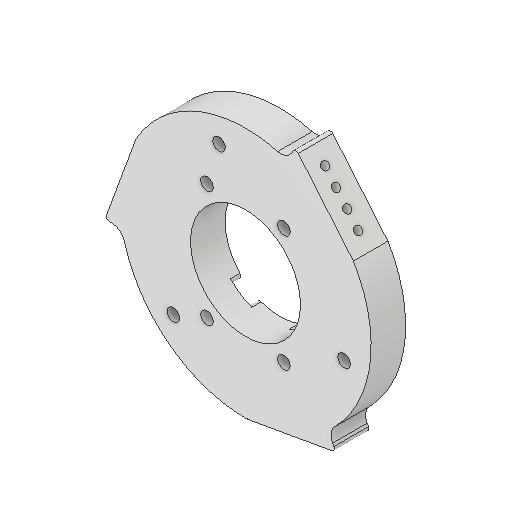
# Autodesk Inventor part: 3DP_ABS_Bowl_Feeder_Base_Plate
Saved by Autodesk Inventor 2025 (Build 290162010, 162A)
## iProperties
Created: 2018-05-26
Part Number: 3DP_ABS_Bowl_Feeder_Base_Plate
Material: ABS Plastic
Document SubType Name: Modeling
Designer: Andrzej
Density: 1.06 g/cm^3
Appearance: Smooth - White
Author: Andrzej
Autodesk Inventor part; units mm, degrees
ref_plane "YZ Plane" through (0, 0, 0) normal (1, 0, 0) x (0, 1, 0)
ref_plane "XZ Plane" through (0, 0, 0) normal (0, 1, 0) x (-1, 0, 0)
ref_plane "XY Plane" through (0, 0, 0) normal (0, 0, 1) x (1, 0, 0)
sketch "Sketch1" plane through (0, 0, 0) normal (0, 0, 1) x (1, 0, 0)
  circle A0 centre (0, 0) radius 40
  circle A1 centre (0, 0) radius 17.5
  dimension "d0" = 80
  dimension "d3" = 35
  constraints: 2 centre point, 2 coincident
  measures "d0" diameter of A0
  measures "d3" diameter of A1
extrude "Extrusion1" add sketch "Sketch1" along normal blind 11
sketch "Sketch2" plane through (0, 0, 11) normal (0, 0, 1) x (1, 0, 0)
  point P0 (0, 0)
  point P1 (-12.25, 18.5)
  point P2 (12.25, 18.5)
  point P3 (-12.25, -18.5)
  point P4 (12.25, -18.5)
  dimension "d4" = 37
  dimension "d5" = 24.5
  dimension "d6" = 18.5
  dimension "d7" = 12.25
  constraints: 2 horizontal alignment, 2 vertical alignment
  measures "d4" distance of point (-12.25, -18.5) point (-12.25, 18.5)
  measures "d5" distance of point (12.25, 18.5) point (-12.25, 18.5)
  measures "d6" vertical distance of point (0, 0) point (-12.25, 18.5)
  measures "d7" horizontal distance of point (0, 0) point (-12.25, 18.5)
hole "Hole1" at (-12.25, 18.5, 11) at (12.25, 18.5, 11) at (-12.25, -18.5, 11) at (12.25, -18.5, 11) direction (0, 0, -1) diameter 4 end through all
sketch "Sketch3" plane through (0, 0, 0) normal (0, 0, -1) x (-1, 0, 0)
  circle A0 centre (12.25, -18.5) radius 2 projected
  circle A1 centre (12.25, 18.5) radius 2 projected
  circle A2 centre (-12.25, 18.5) radius 2 projected
  circle A3 centre (-12.25, -18.5) radius 2 projected
  circle A4 centre (0, 0) radius 17.5 projected
  circle A5 centre (0, 0) radius 40 projected
  line L0 (44.7501, -7.5) -> (39.2906, 7.5)
  line L1 (44.7501, -7.5) -> (95.2438, -7.5) construction
  line L2 (44.7501, -7.5) -> (39.2906, -7.5)
  circle A6 centre (0, 0) radius 40 projected
  line L3 (39.2906, 7.5) -> (34.9192, 19.5102)
  dimension "d16" = 110
  dimension "d17" = 7.5
  dimension "d18" = 7.5
  constraints: 8 end point, 3 point on circle, 2 horizontal, 1 collinear
  measures "d16" angle of L1 L0
  measures "d17" distance from line of point (0, 0) L2
  measures "d18" vertical distance of point (0, 0) L0.end
extrude "Extrusion2" add sketch "Sketch3" against normal up to surface (11 mm away) contours A5 L0 L2
extrude "Extrusion3" cut sketch "Sketch3" against normal up to surface (11 mm away) contours L3 A5 picked at (37.4917, 12.8874)
fillet "Fillet1" radius 4 1 edges at (-39.2906, -7.5, 5.5)
fillet "Fillet1" radius 1 1 edges at (-44.7501, -7.5, 5.5)
sketch "Sketch4" plane through (-34.9192, 19.5102, 0) normal (-0.9396926, 0.3420201, 0) x (0, 0, 1)
  line L0 (11, -27.3155) -> (0, -27.3155) projected
  line L1 (11, -27.3155) -> (11, 0) projected
  line L2 (0, 0) -> (11, 0) projected
  line L3 (0, -27.3155) -> (0, 0) projected
  point P0 (0, -6.3905)
  point P1 (6, -5.4631)
  point P2 (6, -10.9262)
  point P3 (6, -16.3893)
  point P4 (6, -21.8524)
  dimension "d28" = 27.3155
  dimension "d29" = 5.4631
  dimension "d32" = 5.4631
  dimension "d44" = 11
  dimension "d45" = 5
  constraints: 1 vertical, 3 other
  measures "d28" distance between parallel lines of L0 L2
  measures "d29" distance from line of L2 point (6, -5.463)
  measures "d32" distance of point (6, -5.463) point (6, -10.926)
  measures "d44" distance of L2.start L1.end
  measures "d45" distance from line of L1 point (6, -5.463)
hole "Hole2" at (-36.7877, 14.3765, 6) at (-38.6562, 9.2429, 6) at (-40.5247, 4.1093, 6) at (-42.3932, -1.0244, 6) direction (0.9396926, -0.3420201, 0) diameter 2.5 depth 15 tip angle 118
pattern_circular "Circular Pattern2" count 3 over 360 about axis through (0, 0, 0) along (0, 0, 1) of "Extrusion2", "Extrusion3", "Fillet1", "Hole2"
sketch "Sketch5" plane through (0, 0, 11) normal (0, 0, 1) x (1, 0, 0)
  arc A0 (16.7979, 41.4107) -> (15.1658, 41.2679) centre (16.0318, 40.7679) ccw projected
  line L0 (14.7401, 40.5306) -> (15.1658, 41.2679) projected
  arc A1 (10.2509, 38.6642) -> (14.7401, 40.5306) centre (11.276, 42.5306) ccw projected
  arc A2 (10.2509, 38.6642) -> (-34.9192, 19.5102) centre (0, 0) ccw projected
  line L1 (-44.2617, -6.158) -> (-34.9192, 19.5102) projected
  arc A3 (-44.2617, -6.158) -> (-43.322, -7.5) centre (-43.322, -6.5) ccw projected
  line L2 (-42.4706, -7.5) -> (-43.322, -7.5) projected
  arc A4 (-38.6096, -10.4545) -> (-42.4706, -7.5) centre (-42.4706, -11.5) ccw projected
  arc A5 (-38.6096, -10.4545) -> (0.5633, -39.996) centre (0, 0) ccw projected
  line L3 (27.4638, -35.2528) -> (0.5633, -39.996) projected
  arc A6 (27.4638, -35.2528) -> (28.1562, -33.7679) centre (27.2902, -34.2679) ccw projected
  line L4 (27.7305, -33.0306) -> (28.1562, -33.7679) projected
  arc A7 (28.3587, -28.2096) -> (27.7305, -33.0306) centre (31.1946, -31.0306) ccw projected
  arc A8 (28.3587, -28.2096) -> (34.3559, 20.4859) centre (0, 0) ccw projected
  line L5 (16.7979, 41.4107) -> (34.3559, 20.4859) projected
  circle A9 centre (0, 0) radius 17.5 projected
  circle A10 centre (12.25, -18.5) radius 2 projected
  circle A11 centre (12.25, 18.5) radius 2 projected
  circle A12 centre (-12.25, 18.5) radius 2 projected
  circle A13 centre (-12.25, -18.5) radius 2 projected
  line L6 (37.9489, 37.9489) -> (-37.9489, -37.9489)
  line L7 (37.9489, 37.9489) -> (145.2845, 37.9489) construction
  circle A14 centre (0, 0) radius 32.5
  point P0 (-22.981, -22.981)
  dimension "d51" = 65
  dimension "d50" = 135
  constraints: 4 end point, 2 coincident, 1 equal length, 1 horizontal, 1 midpoint, 1 point on line, 3 other
  measures "d50" angle of L6 L7
hole "Hole3" at (-22.981, -22.981, 11) direction (0, 0, -1) diameter 4 end through all
pattern_circular "Circular Pattern3" count 3 over 360 about axis through (0, 0, 0) along (0, 0, 1) of "Hole3"
sketch "Sketch6" plane through (0, 0, 0) normal (0, 0, -1) x (-1, 0, 0)
  circle A0 centre (8.4116, 31.3926) radius 2 projected
  circle A1 centre (-31.3926, -8.4116) radius 2 projected
  circle A2 centre (22.981, -22.981) radius 2 projected
  arc A3 (-15.1658, 41.2679) -> (-16.7979, 41.4107) centre (-16.0318, 40.7679) ccw projected
  line L0 (-16.7979, 41.4107) -> (-34.3559, 20.4859) projected
  arc A4 (-34.3559, 20.4859) -> (-28.3587, -28.2096) centre (0, 0) ccw projected
  arc A5 (-27.7305, -33.0306) -> (-28.3587, -28.2096) centre (-31.1946, -31.0306) ccw projected
  line L1 (-27.7305, -33.0306) -> (-28.1562, -33.7679) projected
  arc A6 (-28.1562, -33.7679) -> (-27.4638, -35.2528) centre (-27.2902, -34.2679) ccw projected
  line L2 (-27.4638, -35.2528) -> (-0.5633, -39.996) projected
  arc A7 (-0.5633, -39.996) -> (38.6096, -10.4545) centre (0, 0) ccw projected
  arc A8 (42.4706, -7.5) -> (38.6096, -10.4545) centre (42.4706, -11.5) ccw projected
  line L3 (42.4706, -7.5) -> (43.322, -7.5) projected
  arc A9 (43.322, -7.5) -> (44.2617, -6.158) centre (43.322, -6.5) ccw projected
  line L4 (44.2617, -6.158) -> (34.9192, 19.5102) projected
  arc A10 (34.9192, 19.5102) -> (-10.2509, 38.6642) centre (0, 0) ccw projected
  arc A11 (-14.7401, 40.5306) -> (-10.2509, 38.6642) centre (-11.276, 42.5306) ccw projected
  line L5 (-14.7401, 40.5306) -> (-15.1658, 41.2679) projected
  circle A12 centre (12.25, -18.5) radius 2 projected
  circle A13 centre (12.25, 18.5) radius 2 projected
  circle A14 centre (-12.25, 18.5) radius 2 projected
  circle A15 centre (-12.25, -18.5) radius 2 projected
  circle A16 centre (0, 0) radius 17.5 projected
  circle A17 centre (12.25, 18.5) radius 5
  circle A18 centre (12.25, -18.5) radius 5
  circle A19 centre (-12.25, 18.5) radius 5
  circle A20 centre (-12.25, -18.5) radius 2 projected
  circle A21 centre (-12.25, -18.5) radius 5
  dimension "d62" = 10
  dimension "d63" = 10
  dimension "d64" = 10
  dimension "d65" = 10
  constraints: 4 centre point, 4 coincident
  measures "d62" diameter of A17
  measures "d63" diameter of A18
  measures "d64" diameter of A19
  measures "d65" diameter of A21
extrude "Extrusion4" cut sketch "Sketch6" against normal blind 3 contours A17 A16 | A16 A17 | A18 A16 | A16 A18 | A19 A16 | A16 A19 | A21 A16 | A16 A21
fillet "Fillet2" radius 1 8 edges at (10.91, -13.6829, 1.5) (8.3382, -15.3858, 1.5) (10.91, 13.6829, 1.5) (8.3382, 15.3858, 1.5) (-8.3382, 15.3858, 1.5) (-10.91, 13.6829, 1.5) (-10.91, -13.6829, 1.5) (-8.3382, -15.3858, 1.5)
equation "\"d6\" = 0.5 * d4"
equation "\"d7\" = 0.5 * d5"
equation "\"d18\" = d17"
equation "\"d29\" = 0.2 * d28"
equation "\"d32\" = d29"
body "Solid1"
